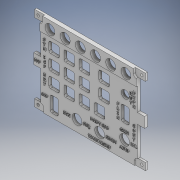
# Autodesk Inventor part: IPC Front Panel
Saved by Autodesk Inventor 2022 (Build 260153000, 153)
## iProperties
Created: 2021-12-31
Part Number: IPC Front Panel
Material: Generic
Document SubType Name: Modeling
Designer: solor
Density: 1 g/cm^3
Appearance: Default
Author: solor
Autodesk Inventor part; units mm, degrees
(part 1 of 2)
ref_plane "YZ Plane" through (0, 0, 0) normal (1, 0, 0) x (0, 1, 0)
ref_plane "XZ Plane" through (0, 0, 0) normal (0, 1, 0) x (-1, 0, 0)
ref_plane "XY Plane" through (0, 0, 0) normal (0, 0, 1) x (1, 0, 0)
sketch "Sketch1" plane through (0, 0, 0) normal (0, 0, 1) x (1, 0, 0)
  line L0 (0.0002, 13.311) -> (12.8002, 13.311) construction
  line L1 (12.8002, 13.311) -> (31.8502, 13.311) construction
  line L2 (31.8502, 13.311) -> (50.9002, 13.311) construction
  line L3 (50.9002, 13.311) -> (69.9502, 13.311) construction
  line L4 (69.9502, 13.311) -> (89.0002, 13.311) construction
  line L5 (89.0002, 13.311) -> (108.0502, 13.311) construction
  line L6 (-24.0572, 0) -> (-24.0572, -106) construction
  line L7 (0.0002, 13.311) -> (-8.9998, 13.311) construction
  line L8 (108.0502, 13.311) -> (120.8502, 13.311) construction
  line L9 (138.0271, 0) -> (138.0271, -10.03) construction
  line L10 (120.8502, 13.311) -> (129.8502, 13.311) construction
  line L11 (-9, 0) -> (-9, -9)
  line L12 (-9, -9) -> (-9, -46.5) construction
  line L13 (-9, -46.5) -> (-9, -59.5)
  line L14 (-9, -59.5) -> (-9, -97) construction
  line L15 (-9, -97) -> (-9, -106)
  line L16 (10, -106) -> (10, -100.81) construction
  line L17 (10, -100.81) -> (10, -81.47) construction
  line L18 (10, -81.47) -> (10, -75.06) construction
  line L19 (10, -75.06) -> (10, -61.92)
  line L20 (10, -61.92) -> (10, -56.04) construction
  line L21 (10, -56.04) -> (10, -42.9)
  line L22 (10, -42.9) -> (10, -37.02) construction
  line L23 (10, -37.02) -> (10, -23.88)
  line L24 (0, -23.88) -> (10, -23.88) construction
  line L25 (10, -23.88) -> (23.08, -23.88)
  line L26 (23.08, -23.88) -> (29.02, -23.88) construction
  line L27 (29.02, -23.88) -> (42.1, -23.88)
  line L28 (42.1, -23.88) -> (48.04, -23.88) construction
  line L29 (48.04, -23.88) -> (61.13, -23.88)
  line L30 (61.13, -23.88) -> (72.63, -23.88) construction
  line L31 (72.63, -23.88) -> (85.71, -23.88)
  line L32 (23.08, -23.88) -> (23.08, -37.02)
  line L33 (23.08, -37.02) -> (10, -37.02)
  line L34 (29.02, -23.88) -> (29.02, -37.02)
  line L35 (29.02, -37.02) -> (42.1, -37.02)
  line L36 (42.1, -37.02) -> (42.1, -23.88)
  line L37 (48.04, -23.88) -> (48.04, -37.02)
  line L38 (48.04, -37.02) -> (61.13, -37.02)
  line L39 (61.13, -37.02) -> (61.13, -23.88)
  line L40 (72.63, -23.88) -> (72.63, -37.02)
  line L41 (72.63, -37.02) -> (85.71, -37.02)
  line L42 (85.71, -37.02) -> (85.71, -23.88)
  line L43 (10, -42.9) -> (23.08, -42.9)
  line L44 (23.08, -42.9) -> (23.08, -56.04)
  line L45 (23.08, -56.04) -> (10, -56.04)
  line L46 (29.02, -42.9) -> (29.02, -56.04)
  line L47 (42.1, -56.04) -> (42.1, -42.9)
  line L48 (29.02, -56.04) -> (42.1, -56.04)
  line L49 (42.1, -42.9) -> (29.02, -42.9)
  line L50 (48.04, -42.9) -> (48.04, -56.04)
  line L51 (48.04, -56.04) -> (61.13, -56.04)
  line L52 (61.13, -56.04) -> (61.13, -42.9)
  line L53 (61.13, -42.9) -> (48.04, -42.9)
  line L54 (72.63, -42.9) -> (72.63, -56.04)
  line L55 (72.63, -56.04) -> (85.71, -56.04)
  line L56 (85.71, -56.04) -> (85.71, -42.9)
  line L57 (85.71, -42.9) -> (72.63, -42.9)
  line L58 (10, -61.92) -> (23.08, -61.92)
  line L59 (23.08, -61.92) -> (23.08, -75.06)
  line L60 (23.08, -75.06) -> (10, -75.06)
  line L61 (29.02, -61.92) -> (42.1, -61.92)
  line L62 (42.1, -61.92) -> (42.1, -75.06)
  line L63 (42.1, -75.06) -> (29.02, -75.06)
  line L64 (29.02, -75.06) -> (29.02, -61.92)
  line L65 (48.04, -61.92) -> (61.13, -61.92)
  line L66 (61.13, -61.92) -> (61.13, -75.06)
  line L67 (61.13, -75.06) -> (48.04, -75.06)
  line L68 (48.04, -75.06) -> (48.04, -61.92)
  line L69 (61.13, -61.92) -> (67.07, -61.92) construction
  line L70 (85.71, -49.47) -> (100.7, -49.47) construction
  line L71 (80.14, -61.92) -> (80.14, -75.06)
  line L72 (80.14, -75.06) -> (67.07, -75.06)
  line L73 (67.07, -75.06) -> (67.07, -61.92)
  line L74 (67.07, -61.92) -> (80.14, -61.92)
  circle A0 centre (12.8, -10.03) radius 6.22
  circle A1 centre (31.85, -10.03) radius 6.22
  circle A2 centre (50.9, -10.03) radius 6.22
  circle A3 centre (69.95, -10.03) radius 6.22
  circle A4 centre (89, -10.03) radius 6.22
  circle A5 centre (108.05, -10.03) radius 6.22
  line L75 (-9, -9) -> (0, -9)
  line L76 (0, -9) -> (0, -46.5)
  line L77 (0, -46.5) -> (-9, -46.5)
  line L78 (-9, -59.5) -> (0, -59.5)
  line L79 (0, -59.5) -> (0, -97)
  line L80 (0, -97) -> (-9, -97)
  line L81 (-9, 0) -> (129.8502, 0)
  line L82 (129.8502, -9) -> (120.8502, -9)
  line L83 (120.8502, -9) -> (120.8502, -46.5)
  line L84 (120.8502, -46.5) -> (129.8502, -46.5)
  line L85 (129.8502, -46.5) -> (129.8502, -59.5)
  line L86 (129.8502, -59.5) -> (120.8502, -59.5)
  line L87 (120.8502, -59.5) -> (120.8502, -97)
  line L88 (120.8502, -97) -> (129.8502, -97)
  line L89 (129.8502, -97) -> (129.8502, -106)
  line L90 (-9, -106) -> (129.8502, -106)
  line L91 (129.8502, 0) -> (129.8502, -9)
  line L92 (118.3416, -106) -> (118.3416, -84.37) construction
  line L93 (118.3416, -84.37) -> (118.3416, -66.16) construction
  line L94 (118.3416, -66.16) -> (118.3416, -46.82) construction
  circle A6 centre (104.8902, -84.37) radius 6.22
  line L95 (120.8502, -117.5908) -> (104.8902, -117.5908) construction
  line L96 (104.8902, -117.5908) -> (73.6502, -117.5908) construction
  line L97 (73.6502, -117.5908) -> (45.1902, -117.5908) construction
  line L98 (45.1902, -117.5908) -> (21.7302, -117.5908) construction
  line L99 (21.7302, -117.5908) -> (11.8502, -117.5908) construction
  line L100 (138.0271, -106) -> (138.0271, -92.18) construction
  circle A7 centre (73.6502, -92.18) radius 6.22
  circle A8 centre (45.1902, -92.18) radius 6.22
  line L101 (21.7302, -100.81) -> (21.7302, -81.47)
  line L102 (21.7302, -81.47) -> (11.8502, -81.47)
  line L103 (11.8502, -81.47) -> (11.8502, -100.81)
  line L104 (11.8502, -100.81) -> (21.7302, -100.81)
  line L105 (100.7, -46.82) -> (110.58, -46.82)
  line L106 (110.58, -46.82) -> (110.58, -66.16)
  line L107 (110.58, -66.16) -> (100.7, -66.16)
  line L108 (100.7, -66.16) -> (100.7, -46.82)
  line L109 (118.3416, -46.82) -> (118.3416, -34.66) construction
  line L110 (118.3416, -34.66) -> (118.3416, -18) construction
  line L111 (120.8502, -18) -> (0, -18)
  circle A9 centre (105.64, -34.66) radius 4.94
  point P0 (0, 0)
  dimension "d1" = 19.05
  dimension "d2" = 19.05
  dimension "d3" = 19.05
  dimension "d4" = 19.05
  dimension "d5" = 19.05
  dimension "d6" = 106
  dimension "d8" = 12.8
  dimension "d10" = 10.03
  dimension "d11" = 9
  dimension "d12" = 9
  dimension "d13" = 37.5
  dimension "d14" = 13
  dimension "d15" = 37.5
  dimension "d16" = 9
  dimension "d17" = 5.19
  dimension "d18" = 19.34
  dimension "d19" = 6.41
  dimension "d20" = 13.14
  dimension "d21" = 5.88
  dimension "d22" = 13.14
  dimension "d23" = 5.88
  dimension "d24" = 13.14
  dimension "d25" = 10
  dimension "d26" = 13.08
  dimension "d27" = 5.94
  dimension "d28" = 13.08
  dimension "d29" = 5.94
  dimension "d30" = 13.09
  dimension "d31" = 11.5
  dimension "d32" = 13.08
  dimension "d33" = 5.94
  dimension "d34" = 14.99
  dimension "d36" = 12.44
  dimension "d37" = 12.44
  dimension "d38" = 12.44
  dimension "d39" = 12.44
  dimension "d40" = 12.44
  dimension "d41" = 12.44
  dimension "d42" = 9
  dimension "d43" = 12.8
  dimension "d44" = 9
  dimension "d45" = 21.63
  dimension "d46" = 18.21
  dimension "d47" = 19.34
  dimension "d49" = 12.44
  dimension "d50" = 15.96
  dimension "d51" = 31.24
  dimension "d52" = 28.46
  dimension "d53" = 23.46
  dimension "d54" = 9.88
  dimension "d55" = 13.82
  dimension "d56" = 12.44
  dimension "d57" = 9.88
  dimension "d58" = 12.16
  dimension "d60" = 16.66
  dimension "d61" = 9.88
  constraints: 224 end point, 84 point on line, 31 perpendicular, 15 horizontal, 13 vertical, 10 centre point, 8 coincident, 4 parallel, 1 midpoint
  measures "d1" distance of L0.end L1.end
  measures "d2" distance of L1.end L2.end
  measures "d3" distance of L2.end L3.end
  measures "d4" distance of L3.end L4.end
  measures "d5" distance of L4.end L5.end
  measures "d6" distance of L6.start L6.end
  measures "d8" distance of L5.end L8.end
  measures "d10" distance of L9.start L9.end
  measures "d11" distance of L8.end L10.end
  measures "d12" distance of L11.start L11.end
  measures "d13" distance of L11.end L12.end
  measures "d14" distance of L12.end L13.end
  measures "d15" distance of L13.end L14.end
  measures "d16" distance of L14.end L15.end
  measures "d17" distance of L16.start L16.end
  measures "d18" distance of L16.end L17.end
  measures "d19" distance of L17.end L18.end
  measures "d20" distance of L18.end L19.end
  measures "d21" distance of L19.end L20.end
  measures "d22" distance of L20.end L21.end
  measures "d23" distance of L21.end L22.end
  measures "d24" distance of L22.end L23.end
  measures "d25" distance of L24.start L24.end
  measures "d26" distance of L24.end L25.end
  measures "d27" distance of L25.end L26.end
  measures "d28" distance of L26.end L27.end
  measures "d29" distance of L27.end L28.end
  measures "d30" distance of L28.end L29.end
  measures "d31" distance of L29.end L30.end
  measures "d32" distance of L30.end L31.end
  measures "d33" distance of L65.end L69.end
  measures "d34" distance of L70.start L70.end
  measures "d36" diameter of A0
  measures "d37" diameter of A1
  measures "d38" diameter of A2
  measures "d39" diameter of A3
  measures "d40" diameter of A4
  measures "d41" diameter of A5
  measures "d42" distance of L0.start L7.end
  measures "d43" distance of L0.start L0.end
  measures "d44" distance of L82.start L82.end
  measures "d45" distance of L92.start L92.end
  measures "d46" distance of L92.end L93.end
  measures "d47" distance of L93.end L94.end
  measures "d49" diameter of A6
  measures "d50" distance of L95.start L95.end
  measures "d51" distance of L95.end L96.end
  measures "d52" distance of L96.end L97.end
  measures "d53" distance of L97.end L98.end
  measures "d54" distance of L98.end L99.end
  measures "d55" distance of L100.start L100.end
  measures "d56" diameter of A7
  measures "d57" distance of L105.start L105.end
  measures "d58" distance of L94.end L109.end
  measures "d60" distance of L109.end L110.end
  measures "d61" diameter of A9
extrude "Extrusion1" add sketch "Sketch1" along normal blind 3.5 contours L111 L83 L84 L85 L86 L87 L88 L89 L90 L15 L80 L79 L78 L13 L77 L76
extrude "Extrusion2" add sketch "Sketch1" along normal blind 5 contours L81 L91 L82 L83 L111 L76 L75 L11
fillet "Fillet1" radius 2 4 edges at (10, -23.88, 1.75) (23.08, -23.88, 1.75) (10, -37.02, 1.75) (23.08, -37.02, 1.75)
fillet "Fillet2" radius 2 12 edges at (29.02, -23.88, 1.75) (29.02, -37.02, 1.75) (42.1, -37.02, 1.75) (42.1, -23.88, 1.75) (48.04, -23.88, 1.75) (48.04, -37.02, 1.75) (61.13, -37.02, 1.75) (61.13, -23.88, 1.75) (72.63, -23.88, 1.75) (72.63, -37.02, 1.75) (85.71, -37.02, 1.75) (85.71, -23.88, 1.75)
fillet "Fillet3" radius 2 20 edges at (10, -42.9, 1.75) (10, -56.04, 1.75) (23.08, -56.04, 1.75) (23.08, -42.9, 1.75) (29.02, -42.9, 1.75) (29.02, -56.04, 1.75) (42.1, -56.04, 1.75) (42.1, -42.9, 1.75) (48.04, -42.9, 1.75) (48.04, -56.04, 1.75) (61.13, -56.04, 1.75) (61.13, -42.9, 1.75) (72.63, -42.9, 1.75) (72.63, -56.04, 1.75) (85.71, -56.04, 1.75) (85.71, -42.9, 1.75) (100.7, -46.82, 1.75) (100.7, -66.16, 1.75) (110.58, -66.16, 1.75) (110.58, -46.82, 1.75)
fillet "Fillet4" radius 2 20 edges at (10, -75.06, 1.75) (10, -61.92, 1.75) (23.08, -61.92, 1.75) (23.08, -75.06, 1.75) (29.02, -75.06, 1.75) (29.02, -61.92, 1.75) (42.1, -61.92, 1.75) (42.1, -75.06, 1.75) (48.04, -75.06, 1.75) (48.04, -61.92, 1.75) (61.13, -61.92, 1.75) (61.13, -75.06, 1.75) (67.07, -75.06, 1.75) (67.07, -61.92, 1.75) (80.14, -75.06, 1.75) (80.14, -61.92, 1.75) (21.7302, -100.81, 1.75) (11.8502, -100.81, 1.75) (11.8502, -81.47, 1.75) (21.7302, -81.47, 1.75)
sketch "Sketch2" plane through (0, 0, 5) normal (0, 0, 1) x (1, 0, 0)
  line L0 (-9, -9) -> (0, -9) projected
  line L1 (3.5, -5.5828) -> (3.5, 0)
  line L2 (129.8502, 0) -> (-9, 0) projected
  arc A0 (0, -9) -> (3.501, -5.499) centre (0, -5.499) ccw
  line L3 (0, -9) -> (0, -5.499) construction
  line L4 (3.501, -5.499) -> (0, -5.499) construction
  line L5 (60.4251, 0) -> (60.4251, -11.5403)
  line L6 (-9, -106) -> (129.8502, -106) projected
  line L7 (-42.3083, 0) -> (-42.3083, -53)
  line L8 (-42.3083, -53) -> (-15.0047, -53)
  line L9 (3.5, 0) -> (-9, 0)
  line L10 (-9, 0) -> (-9, -9) projected
  line L11 (-9, 0) -> (-9, -9)
  line L12 (0, -9) -> (0, -46.5) projected
  line L13 (-9, -9) -> (0, -9)
  circle A1 centre (-4.5, -4.5) radius 1.65
  line L14 (129.8502, -9) -> (120.8502, -9)
  line L15 (117.3502, -5.5828) -> (117.3502, 0)
  arc A2 (117.3492, -5.499) -> (120.8502, -9) centre (120.8502, -5.499) ccw
  line L16 (163.1585, -53) -> (135.855, -53)
  line L17 (117.3502, 0) -> (129.8502, 0)
  line L18 (129.8502, 0) -> (129.8502, -9)
  circle A3 centre (125.3502, -4.5) radius 1.65
  line L19 (-9, -97) -> (0, -97)
  line L20 (3.5, -100.4172) -> (3.5, -106)
  line L21 (129.8502, -106) -> (-9, -106)
  arc A4 (3.501, -100.501) -> (0, -97) centre (0, -100.501) ccw
  line L22 (-9, -106) -> (-9, -97)
  circle A5 centre (-4.5, -101.5) radius 1.65
  circle A6 centre (125.3502, -101.5) radius 1.65
  line L23 (129.8502, -97) -> (120.8502, -97)
  line L24 (129.8502, -106) -> (129.8502, -97)
  line L25 (117.3502, -100.4172) -> (117.3502, -106)
  arc A7 (120.8502, -97) -> (117.3492, -100.501) centre (120.8502, -100.501) ccw
  point P0 (0, 0)
  dimension "d71" = 90
  dimension "d72" = 53
  dimension "d73" = 3.3
  constraints: 42 end point, 23 symmetric about line, 12 point on circle, 8 centre point, 3 point on line, 3 vertical, 2 collinear, 1 horizontal, 1 midpoint, 1 perpendicular, 1 tangent, 6 other
  measures "d71" angle of L3 L4
  measures "d72" distance of L7.start L7.end
  measures "d73" diameter of A1
extrude "Extrusion3" cut sketch "Sketch2" against normal blind 2.5
extrude "Extrusion4" cut sketch "Sketch2" against normal blind 18.1375 contours A1 | A3 | A5 | A6
sketch "Sketch3" plane through (0, 0, 3.5) normal (0, 0, 1) x (1, 0, 0)
  line L0 (3.5998, -42.9233) -> (6.4002, -42.9233) construction
  line L1 (6.4002, -42.9233) -> (6.4002, -56.0167) construction
  line L2 (6.4002, -56.0167) -> (3.5998, -56.0167) construction
  line L3 (3.5998, -56.0167) -> (3.5998, -42.9233) construction
  line L4 (3.4775, -61.9433) -> (6.5225, -61.9433) construction
  line L5 (6.5225, -61.9433) -> (6.5225, -75.0367) construction
  line L6 (6.5225, -75.0367) -> (3.4775, -75.0367) construction
  line L7 (3.4775, -75.0367) -> (3.4775, -61.9433) construction
  line L8 (-8.5522, -51.4107) -> (-0.4478, -51.4107) construction
  line L9 (-0.4478, -51.4107) -> (-0.4478, -54.5893) construction
  line L10 (-0.4478, -54.5893) -> (-8.5522, -54.5893) construction
  line L11 (-8.5522, -54.5893) -> (-8.5522, -51.4107) construction
  line L12 (0.9302, -84.0431) -> (9.0347, -84.0431) construction
  line L13 (9.0347, -84.0431) -> (9.0347, -87.2216) construction
  line L14 (9.0347, -87.2216) -> (0.9302, -87.2216) construction
  line L15 (0.9302, -87.2216) -> (0.9302, -84.0431) construction
  line L16 (28.3443, -90.655) -> (37.1902, -90.655) construction
  line L17 (37.1902, -90.655) -> (37.1902, -93.705) construction
  line L18 (37.1902, -93.705) -> (28.3443, -93.705) construction
  line L19 (28.3443, -93.705) -> (28.3443, -90.655) construction
  line L20 (53.1902, -90.1903) -> (61.6581, -90.1903) construction
  line L21 (61.6581, -90.1903) -> (61.6581, -94.1697) construction
  line L22 (61.6581, -94.1697) -> (53.1902, -94.1697) construction
  line L23 (53.1902, -94.1697) -> (53.1902, -90.1903) construction
  line L24 (62.1843, -80.3317) -> (85.1162, -80.3317) construction
  line L25 (85.1162, -80.3317) -> (85.1162, -84.18) construction
  line L26 (85.1162, -84.18) -> (62.1843, -84.18) construction
  line L27 (62.1843, -84.18) -> (62.1843, -80.3317) construction
  line L28 (59.5891, -100.18) -> (87.7114, -100.18) construction
  line L29 (87.7114, -100.18) -> (87.7114, -103.3388) construction
  line L30 (87.7114, -103.3388) -> (59.5891, -103.3388) construction
  line L31 (59.5891, -103.3388) -> (59.5891, -100.18) construction
  line L32 (81.6502, -90.5907) -> (94.9056, -90.5907) construction
  line L33 (94.9056, -90.5907) -> (94.9056, -93.7693) construction
  line L34 (94.9056, -93.7693) -> (81.6502, -93.7693) construction
  line L35 (81.6502, -93.7693) -> (81.6502, -90.5907) construction
  line L36 (99.2623, -73.1964) -> (110.5182, -73.1964) construction
  line L37 (110.5182, -73.1964) -> (110.5182, -76.37) construction
  line L38 (110.5182, -76.37) -> (99.2623, -76.37) construction
  line L39 (99.2623, -76.37) -> (99.2623, -73.1964) construction
  line L40 (99.0053, -92.37) -> (110.7752, -92.37) construction
  line L41 (110.7752, -92.37) -> (110.7752, -95.5485) construction
  line L42 (110.7752, -95.5485) -> (99.0053, -95.5485) construction
  line L43 (99.0053, -95.5485) -> (99.0053, -92.37) construction
  line L44 (112.8902, -82.845) -> (120.5202, -82.845) construction
  line L45 (120.5202, -82.845) -> (120.5202, -85.895) construction
  line L46 (120.5202, -85.895) -> (112.8902, -85.895) construction
  line L47 (112.8902, -85.895) -> (112.8902, -82.845) construction
  line L48 (115.4917, -61.3021) -> (118.7246, -61.3021) construction
  line L49 (118.7246, -61.3021) -> (118.7246, -79.4767) construction
  line L50 (118.7246, -79.4767) -> (115.4917, -79.4767) construction
  line L51 (115.4917, -79.4767) -> (115.4917, -61.3021) construction
  line L52 (95.6549, -47.4324) -> (98.7, -47.4324) construction
  line L53 (98.7, -47.4324) -> (98.7, -65.5476) construction
  line L54 (98.7, -65.5476) -> (95.6549, -65.5476) construction
  line L55 (95.6549, -65.5476) -> (95.6549, -47.4324) construction
  line L56 (115.64, -25.6024) -> (118.8161, -25.6024) construction
  line L57 (118.8161, -25.6024) -> (118.8161, -43.7176) construction
  line L58 (118.8161, -43.7176) -> (115.64, -43.7176) construction
  line L59 (115.64, -43.7176) -> (115.64, -25.6024) construction
  line L60 (111.64, -28.1133) -> (114.6851, -28.1133) construction
  line L61 (114.6851, -28.1133) -> (114.6851, -41.2067) construction
  line L62 (114.6851, -41.2067) -> (111.64, -41.2067) construction
  line L63 (111.64, -41.2067) -> (111.64, -28.1133) construction
  line L64 (10, -35.02) -> (10, -25.88) projected
  line L65 (0, -9) -> (0, -46.5) projected
  line L66 (0, -19.838) -> (10, -19.838)
  line L67 (3.1265, -23.8761) -> (6.8735, -23.8761) construction
  line L68 (6.8735, -23.8761) -> (6.8735, -37.0239) construction
  line L69 (6.8735, -37.0239) -> (3.1265, -37.0239) construction
  line L70 (3.1265, -37.0239) -> (3.1265, -23.8761) construction
  line L71 (10, -54.04) -> (10, -44.9) projected
  line L72 (10, -73.06) -> (10, -63.92) projected
  line L73 (-9, -59.5) -> (0, -59.5) projected
  line L74 (-9, -46.5) -> (-9, -59.5) projected
  circle A0 centre (45.1902, -92.18) radius 6.22 construction
  circle A1 centre (73.6502, -92.18) radius 6.22 construction
  line L75 (45.1902, -92.18) -> (37.1902, -92.18) construction
  line L76 (45.1902, -92.18) -> (53.1902, -92.18) construction
  line L77 (73.6502, -92.18) -> (73.6502, -84.18) construction
  line L78 (73.6502, -92.18) -> (81.6502, -92.18) construction
  line L79 (73.6502, -92.18) -> (73.6502, -100.18) construction
  circle A2 centre (104.8902, -84.37) radius 6.22 construction
  line L80 (104.8902, -84.37) -> (112.8902, -84.37) construction
  line L81 (104.8902, -84.37) -> (104.8902, -76.37) construction
  line L82 (104.8902, -84.37) -> (104.8902, -92.37) construction
  line L83 (100.7, -64.16) -> (100.7, -48.82) construction
  circle A3 centre (105.64, -34.66) radius 4.94 construction
  spline S0 degree 2 poles (-5.4602, -53) (-5.4602, -53.7415) (-6.2512, -54.5893) (-6.9383, -54.5893) knots 0 0 0 1 2 2 2
  spline S1 degree 2 poles (-6.9383, -54.5893) (-7.6279, -54.5893) (-8.4138, -53.7316) (-8.4138, -53) knots 0 0 0 1 2 2 2
  spline S2 degree 2 poles (-8.4138, -53) (-8.4138, -52.2659) (-7.6279, -51.4107) (-6.9383, -51.4107) knots 0 0 0 1 2 2 2
  spline S3 degree 2 poles (-6.9383, -51.4107) (-6.2512, -51.4107) (-5.4602, -52.261) (-5.4602, -53) knots 0 0 0 1 2 2 2
  spline S4 degree 2 poles (-6.2512, -53) (-6.2512, -52.7256) (-6.3624, -52.3425) (-6.4588, -52.2214) knots 0 0 0 1 2 2 2
  spline S5 degree 2 poles (-6.4588, -52.2214) (-6.5552, -52.0954) (-6.8023, -51.9866) (-6.9358, -51.9866) knots 0 0 0 1 2 2 2
  spline S6 degree 2 poles (-6.9358, -51.9866) (-7.0767, -51.9866) (-7.3065, -52.088) (-7.4128, -52.2165) knots 0 0 0 1 2 2 2
  spline S7 degree 2 poles (-7.4128, -52.2165) (-7.5067, -52.3351) (-7.6229, -52.7281) (-7.6229, -53) knots 0 0 0 1 2 2 2
  spline S8 degree 2 poles (-7.6229, -53) (-7.6229, -53.2818) (-7.5117, -53.6525) (-7.4153, -53.7786) knots 0 0 0 1 2 2 2
  spline S9 degree 2 poles (-7.4153, -53.7786) (-7.3189, -53.9046) (-7.0693, -54.0134) (-6.9358, -54.0134) knots 0 0 0 1 2 2 2
  spline S10 degree 2 poles (-6.9358, -54.0134) (-6.7999, -54.0134) (-6.5478, -53.8972) (-6.4563, -53.7736) knots 0 0 0 1 2 2 2
  spline S11 degree 2 poles (-6.4563, -53.7736) (-6.3574, -53.6402) (-6.2512, -53.2867) (-6.2512, -53) knots 0 0 0 1 2 2 2
  line L84 (-2.9639, -52.0558) -> (-4.2442, -52.0558)
  line L85 (-4.2442, -52.0558) -> (-4.2442, -52.6317)
  line L86 (-4.2442, -52.6317) -> (-3.0652, -52.6317)
  line L87 (-3.0652, -52.6317) -> (-3.0652, -53.2126)
  line L88 (-3.0652, -53.2126) -> (-4.2442, -53.2126)
  line L89 (-4.2442, -53.2126) -> (-4.2442, -54.525)
  line L90 (-4.2442, -54.525) -> (-5.0054, -54.525)
  line L91 (-5.0054, -54.525) -> (-5.0054, -51.475)
  line L92 (-5.0054, -51.475) -> (-2.9639, -51.475)
  line L93 (-2.9639, -51.475) -> (-2.9639, -52.0558)
  line L94 (-0.5268, -52.0558) -> (-1.8072, -52.0558)
  line L95 (-1.8072, -52.0558) -> (-1.8072, -52.6317)
  line L96 (-1.8072, -52.6317) -> (-0.6282, -52.6317)
  line L97 (-0.6282, -52.6317) -> (-0.6282, -53.2126)
  line L98 (-0.6282, -53.2126) -> (-1.8072, -53.2126)
  line L99 (-1.8072, -53.2126) -> (-1.8072, -54.525)
  line L100 (-1.8072, -54.525) -> (-2.5684, -54.525)
  line L101 (-2.5684, -54.525) -> (-2.5684, -51.475)
  line L102 (-2.5684, -51.475) -> (-0.5268, -51.475)
  line L103 (-0.5268, -51.475) -> (-0.5268, -52.0558)
  line L104 (5.4338, -45.9733) -> (3.7926, -45.9733)
  line L105 (3.7926, -45.9733) -> (3.7926, -45.4419)
  line L106 (3.7926, -45.4419) -> (4.2301, -45.4419)
  line L107 (4.2301, -45.4419) -> (4.2301, -43.4547)
  line L108 (4.2301, -43.4547) -> (3.7926, -43.4547)
  line L109 (3.7926, -43.4547) -> (3.7926, -42.9233)
  line L110 (3.7926, -42.9233) -> (5.4338, -42.9233)
  line L111 (5.4338, -42.9233) -> (5.4338, -43.4547)
  line L112 (5.4338, -43.4547) -> (4.9963, -43.4547)
  line L113 (4.9963, -43.4547) -> (4.9963, -45.4419)
  line L114 (4.9963, -45.4419) -> (5.4338, -45.4419)
  line L115 (5.4338, -45.4419) -> (5.4338, -45.9733)
  spline S12 degree 2 poles (5.2311, -51.0543) (4.544, -51.0543) (3.7382, -50.2238) (3.7382, -49.4725) knots 0 0 0 1 2 2 2
  spline S13 degree 2 poles (3.7382, -49.4725) (3.7382, -48.7483) (4.5465, -47.8857) (5.2336, -47.8857) knots 0 0 0 1 2 2 2
  spline S14 degree 2 poles (5.2336, -47.8857) (5.414, -47.8857) (5.7057, -47.9277) (5.8391, -47.9623) knots 0 0 0 1 2 2 2
  spline S15 degree 2 poles (5.8391, -47.9623) (5.9429, -47.9944) (6.1876, -48.1007) (6.2642, -48.1403) knots 0 0 0 1 2 2 2
  line L116 (6.2642, -48.1403) -> (6.2642, -48.8669)
  line L117 (6.2642, -48.8669) -> (6.1876, -48.8669)
  spline S16 degree 2 poles (6.1876, -48.8669) (6.1308, -48.8175) (5.9627, -48.6791) (5.8564, -48.6148) knots 0 0 0 1 2 2 2
  spline S17 degree 2 poles (5.8564, -48.6148) (5.7501, -48.5481) (5.4956, -48.4566) (5.3547, -48.4566) knots 0 0 0 1 2 2 2
  spline S18 degree 2 poles (5.3547, -48.4566) (5.1891, -48.4566) (4.9147, -48.5604) (4.7887, -48.6914) knots 0 0 0 1 2 2 2
  spline S19 degree 2 poles (4.7887, -48.6914) (4.675, -48.8076) (4.5292, -49.2055) (4.5292, -49.4749) knots 0 0 0 1 2 2 2
  spline S20 degree 2 poles (4.5292, -49.4749) (4.5292, -49.7592) (4.6799, -50.1472) (4.8035, -50.2659) knots 0 0 0 1 2 2 2
  spline S21 degree 2 poles (4.8035, -50.2659) (4.9221, -50.382) (5.2138, -50.4834) (5.3596, -50.4834) knots 0 0 0 1 2 2 2
  spline S22 degree 2 poles (5.3596, -50.4834) (5.5104, -50.4834) (5.7847, -50.382) (5.8787, -50.3202) knots 0 0 0 1 2 2 2
  spline S23 degree 2 poles (5.8787, -50.3202) (5.9825, -50.2585) (6.1382, -50.1275) (6.195, -50.0756) knots 0 0 0 1 2 2 2
  line L118 (6.195, -50.0756) -> (6.2642, -50.0756)
  line L119 (6.2642, -50.0756) -> (6.2642, -50.7923)
  spline S24 degree 2 poles (6.2642, -50.7923) (6.1802, -50.8319) (5.9602, -50.9307) (5.8416, -50.9653) knots 0 0 0 1 2 2 2
  spline S25 degree 2 poles (5.8416, -50.9653) (5.6982, -51.0098) (5.4486, -51.0543) (5.2311, -51.0543) knots 0 0 0 1 2 2 2
  spline S26 degree 2 poles (6.2618, -53.9282) (6.2618, -54.1408) (6.1258, -54.5263) (5.9998, -54.6549) knots 0 0 0 1 2 2 2
  spline S27 degree 2 poles (5.9998, -54.6549) (5.9232, -54.7364) (5.7353, -54.8699) (5.6241, -54.9169) knots 0 0 0 1 2 2 2
  spline S28 degree 2 poles (5.6241, -54.9169) (5.5104, -54.9638) (5.2459, -55.0182) (5.0828, -55.0182) knots 0 0 0 1 2 2 2
  line L120 (5.0828, -55.0182) -> (4.6824, -55.0182)
  line L121 (4.6824, -55.0182) -> (4.6824, -56.0167)
  line L122 (4.6824, -56.0167) -> (3.9162, -56.0167)
  line L123 (3.9162, -56.0167) -> (3.9162, -52.9667)
  line L124 (3.9162, -52.9667) -> (5.1001, -52.9667)
  spline S29 degree 2 poles (5.1001, -52.9667) (5.3621, -52.9667) (5.7452, -53.0631) (5.9009, -53.1669) knots 0 0 0 1 2 2 2
  spline S30 degree 2 poles (5.9009, -53.1669) (6.0739, -53.2831) (6.2618, -53.6637) (6.2618, -53.9282) knots 0 0 0 1 2 2 2
  spline S31 degree 2 poles (5.4758, -53.948) (5.4758, -53.817) (5.3522, -53.6316) (5.2682, -53.597) knots 0 0 0 1 2 2 2
  spline S32 degree 2 poles (5.2682, -53.597) (5.1594, -53.5501) (4.9617, -53.5352) (4.7911, -53.5352) knots 0 0 0 1 2 2 2
  line L125 (4.7911, -53.5352) -> (4.6824, -53.5352)
  line L126 (4.6824, -53.5352) -> (4.6824, -54.4497)
  line L127 (4.6824, -54.4497) -> (4.7368, -54.4497)
  spline S33 degree 2 poles (4.7368, -54.4497) (4.8431, -54.4497) (5.0358, -54.4448) (5.1075, -54.4324) knots 0 0 0 1 2 2 2
  spline S34 degree 2 poles (5.1075, -54.4324) (5.1693, -54.4225) (5.3052, -54.3632) (5.3423, -54.3261) knots 0 0 0 1 2 2 2
  spline S35 degree 2 poles (5.3423, -54.3261) (5.4214, -54.252) (5.4758, -54.0864) (5.4758, -53.948) knots 0 0 0 1 2 2 2
  spline S36 degree 2 poles (4.3846, -27.0348) (4.0336, -27.0348) (3.5047, -26.8989) (3.2773, -26.8) knots 0 0 0 1 2 2 2
  line L128 (3.2773, -26.8) -> (3.2773, -26.0734)
  line L129 (3.2773, -26.0734) -> (3.3465, -26.0734)
  spline S37 degree 2 poles (3.3465, -26.0734) (3.5763, -26.2686) (4.1275, -26.4787) (4.387, -26.4787) knots 0 0 0 1 2 2 2
  spline S38 degree 2 poles (4.387, -26.4787) (4.4538, -26.4787) (4.6688, -26.449) (4.7331, -26.4194) knots 0 0 0 1 2 2 2
  spline S39 degree 2 poles (4.7331, -26.4194) (4.8122, -26.3848) (4.9234, -26.2587) (4.9234, -26.1574) knots 0 0 0 1 2 2 2
  spline S40 degree 2 poles (4.9234, -26.1574) (4.9234, -26.0412) (4.7429, -25.8979) (4.6194, -25.8657) knots 0 0 0 1 2 2 2
  spline S41 degree 2 poles (4.6194, -25.8657) (4.4637, -25.8237) (4.1102, -25.752) (3.9545, -25.6977) knots 0 0 0 1 2 2 2
  spline S42 degree 2 poles (3.9545, -25.6977) (3.6011, -25.5741) (3.2946, -25.1514) (3.2946, -24.8351) knots 0 0 0 1 2 2 2
  spline S43 degree 2 poles (3.2946, -24.8351) (3.2946, -24.4075) (4.0188, -23.8761) (4.5625, -23.8761) knots 0 0 0 1 2 2 2
  spline S44 degree 2 poles (4.5625, -23.8761) (4.8344, -23.8761) (5.3732, -23.9873) (5.5858, -24.0812) knots 0 0 0 1 2 2 2
  line L130 (5.5858, -24.0812) -> (5.5858, -24.7782)
  line L131 (5.5858, -24.7782) -> (5.519, -24.7782)
  spline S45 degree 2 poles (5.519, -24.7782) (5.3485, -24.6324) (4.8591, -24.4322) (4.6021, -24.4322) knots 0 0 0 1 2 2 2
  spline S46 degree 2 poles (4.6021, -24.4322) (4.5007, -24.4322) (4.3425, -24.4618) (4.2536, -24.5014) knots 0 0 0 1 2 2 2
  spline S47 degree 2 poles (4.2536, -24.5014) (4.1819, -24.5335) (4.0781, -24.662) (4.0781, -24.7411) knots 0 0 0 1 2 2 2
  spline S48 degree 2 poles (4.0781, -24.7411) (4.0781, -24.8598) (4.2437, -24.9957) (4.481, -25.0501) knots 0 0 0 1 2 2 2
  spline S49 degree 2 poles (4.481, -25.0501) (4.6342, -25.0847) (4.9184, -25.1514) (5.0816, -25.2083) knots 0 0 0 1 2 2 2
  spline S50 degree 2 poles (5.0816, -25.2083) (5.3979, -25.3244) (5.7069, -25.71) (5.7069, -26.0264) knots 0 0 0 1 2 2 2
  spline S51 degree 2 poles (5.7069, -26.0264) (5.7069, -26.4812) (4.9926, -27.0348) (4.3846, -27.0348) knots 0 0 0 1 2 2 2
  line L132 (5.9788, -28.9522) -> (4.9259, -30.7293)
  line L133 (4.9259, -30.7293) -> (4.9259, -32.0022)
  line L134 (4.9259, -32.0022) -> (4.1596, -32.0022)
  line L135 (4.1596, -32.0022) -> (4.1596, -30.7664)
  line L136 (4.1596, -30.7664) -> (3.0894, -28.9522)
  line L137 (3.0894, -28.9522) -> (3.9619, -28.9522)
  line L138 (3.9619, -28.9522) -> (4.5576, -30.0397)
  line L139 (4.5576, -30.0397) -> (5.1335, -28.9522)
  line L140 (5.1335, -28.9522) -> (5.9788, -28.9522)
  line L141 (6.5571, -37.0239) -> (5.7959, -37.0239)
  line L142 (5.7959, -37.0239) -> (5.7959, -35.0021)
  line L143 (5.7959, -35.0021) -> (5.2422, -36.3072)
  line L144 (5.2422, -36.3072) -> (4.7182, -36.3072)
  line L145 (4.7182, -36.3072) -> (4.1646, -35.0021)
  line L146 (4.1646, -35.0021) -> (4.1646, -37.0239)
  line L147 (4.1646, -37.0239) -> (3.4429, -37.0239)
  line L148 (3.4429, -37.0239) -> (3.4429, -33.9739)
  line L149 (3.4429, -33.9739) -> (4.3252, -33.9739)
  line L150 (4.3252, -33.9739) -> (5.0025, -35.4792)
  line L151 (5.0025, -35.4792) -> (5.6748, -33.9739)
  line L152 (5.6748, -33.9739) -> (6.5571, -33.9739)
  line L153 (6.5571, -33.9739) -> (6.5571, -37.0239)
  spline S52 degree 2 poles (6.2309, -64.059) (6.2309, -64.2864) (6.0579, -64.6299) (5.9145, -64.7436) knots 0 0 0 1 2 2 2
  spline S53 degree 2 poles (5.9145, -64.7436) (5.7415, -64.8796) (5.3312, -64.9933) (5.0124, -64.9933) knots 0 0 0 1 2 2 2
  line L154 (5.0124, -64.9933) -> (3.7938, -64.9933)
  line L155 (3.7938, -64.9933) -> (3.7938, -61.9433)
  line L156 (3.7938, -61.9433) -> (4.869, -61.9433)
  spline S54 degree 2 poles (4.869, -61.9433) (5.2051, -61.9433) (5.5512, -61.9952) (5.7019, -62.0767) knots 0 0 0 1 2 2 2
  spline S55 degree 2 poles (5.7019, -62.0767) (5.8675, -62.1632) (6.0282, -62.4598) (6.0282, -62.6526) knots 0 0 0 1 2 2 2
  spline S56 degree 2 poles (6.0282, -62.6526) (6.0282, -62.8751) (5.8058, -63.2236) (5.608, -63.3051) knots 0 0 0 1 2 2 2
  line L157 (5.608, -63.3051) -> (5.608, -63.32)
  spline S57 degree 2 poles (5.608, -63.32) (5.8923, -63.3793) (6.2309, -63.7476) (6.2309, -64.059) knots 0 0 0 1 2 2 2
  spline S58 degree 2 poles (5.44, -64.0466) (5.44, -63.9033) (5.3263, -63.7426) (5.2126, -63.7006) knots 0 0 0 1 2 2 2
  spline S59 degree 2 poles (5.2126, -63.7006) (5.1434, -63.6734) (4.8987, -63.6685) (4.696, -63.6685) knots 0 0 0 1 2 2 2
  line L158 (4.696, -63.6685) -> (4.5551, -63.6685)
  line L159 (4.5551, -63.6685) -> (4.5551, -64.4371)
  line L160 (4.5551, -64.4371) -> (4.5971, -64.4371)
  spline S60 degree 2 poles (4.5971, -64.4371) (4.8937, -64.4371) (5.1211, -64.4297) (5.2397, -64.3778) knots 0 0 0 1 2 2 2
  spline S61 degree 2 poles (5.2397, -64.3778) (5.3436, -64.3309) (5.44, -64.1578) (5.44, -64.0466) knots 0 0 0 1 2 2 2
  spline S62 degree 2 poles (5.2496, -62.8034) (5.2496, -62.7292) (5.173, -62.5735) (5.0939, -62.5389) knots 0 0 0 1 2 2 2
  spline S63 degree 2 poles (5.0939, -62.5389) (5.0198, -62.5043) (4.8122, -62.4994) (4.607, -62.4994) knots 0 0 0 1 2 2 2
  line L161 (4.607, -62.4994) -> (4.5551, -62.4994)
  line L162 (4.5551, -62.4994) -> (4.5551, -63.1469)
  line L163 (4.5551, -63.1469) -> (4.6515, -63.1469)
  spline S64 degree 2 poles (4.6515, -63.1469) (4.8468, -63.1469) (5.0049, -63.1395) (5.089, -63.1) knots 0 0 0 1 2 2 2
  spline S65 degree 2 poles (5.089, -63.1) (5.1804, -63.0555) (5.2496, -62.9047) (5.2496, -62.8034) knots 0 0 0 1 2 2 2
  line L164 (6.6115, -70.015) -> (5.6797, -70.015)
  line L165 (5.6797, -70.015) -> (4.8319, -68.8953)
  line L166 (4.8319, -68.8953) -> (4.5551, -68.8953)
  line L167 (4.5551, -68.8953) -> (4.5551, -70.015)
  line L168 (4.5551, -70.015) -> (3.7938, -70.015)
  line L169 (3.7938, -70.015) -> (3.7938, -66.965)
  line L170 (3.7938, -66.965) -> (5.0198, -66.965)
  spline S66 degree 2 poles (5.0198, -66.965) (5.2744, -66.965) (5.65, -67.0293) (5.8107, -67.1281) knots 0 0 0 1 2 2 2
  spline S67 degree 2 poles (5.8107, -67.1281) (5.9738, -67.2319) (6.1666, -67.5557) (6.1666, -67.8029) knots 0 0 0 1 2 2 2
  spline S68 degree 2 poles (6.1666, -67.8029) (6.1666, -68.1514) (5.8502, -68.5889) (5.5858, -68.7174) knots 0 0 0 1 2 2 2
  line L171 (5.5858, -68.7174) -> (6.6115, -70.015)
  spline S69 degree 2 poles (5.3806, -67.8993) (5.3806, -67.7831) (5.2917, -67.6175) (5.1903, -67.573) knots 0 0 0 1 2 2 2
  spline S70 degree 2 poles (5.1903, -67.573) (5.1186, -67.5434) (4.9432, -67.5261) (4.8122, -67.5261) knots 0 0 0 1 2 2 2
  line L172 (4.8122, -67.5261) -> (4.5551, -67.5261)
  line L173 (4.5551, -67.5261) -> (4.5551, -68.3466)
  line L174 (4.5551, -68.3466) -> (4.7751, -68.3466)
  spline S71 degree 2 poles (4.7751, -68.3466) (4.9333, -68.3466) (5.1582, -68.3071) (5.2348, -68.2453) knots 0 0 0 1 2 2 2
  spline S72 degree 2 poles (5.2348, -68.2453) (5.309, -68.186) (5.3806, -68.0278) (5.3806, -67.8993) knots 0 0 0 1 2 2 2
  line L175 (4.3796, -75.0367) -> (4.3796, -72.5676)
  line L176 (4.3796, -72.5676) -> (3.4775, -72.5676)
  line L177 (3.4775, -72.5676) -> (3.4775, -71.9867)
  line L178 (3.4775, -71.9867) -> (6.048, -71.9867)
  line L179 (6.048, -71.9867) -> (6.048, -72.5676)
  line L180 (6.048, -72.5676) -> (5.1458, -72.5676)
  line L181 (5.1458, -72.5676) -> (5.1458, -75.0367)
  line L182 (5.1458, -75.0367) -> (4.3796, -75.0367)
  spline S73 degree 2 poles (4.0222, -85.6324) (4.0222, -86.3739) (3.2313, -87.2216) (2.5442, -87.2216) knots 0 0 0 1 2 2 2
  spline S74 degree 2 poles (2.5442, -87.2216) (1.8546, -87.2216) (1.0686, -86.364) (1.0686, -85.6324) knots 0 0 0 1 2 2 2
  spline S75 degree 2 poles (1.0686, -85.6324) (1.0686, -84.8983) (1.8546, -84.0431) (2.5442, -84.0431) knots 0 0 0 1 2 2 2
  spline S76 degree 2 poles (2.5442, -84.0431) (3.2313, -84.0431) (4.0222, -84.8934) (4.0222, -85.6324) knots 0 0 0 1 2 2 2
  spline S77 degree 2 poles (3.2313, -85.6324) (3.2313, -85.358) (3.1201, -84.9749) (3.0237, -84.8538) knots 0 0 0 1 2 2 2
  spline S78 degree 2 poles (3.0237, -84.8538) (2.9273, -84.7278) (2.6801, -84.619) (2.5466, -84.619) knots 0 0 0 1 2 2 2
  spline S79 degree 2 poles (2.5466, -84.619) (2.4058, -84.619) (2.1759, -84.7203) (2.0696, -84.8489) knots 0 0 0 1 2 2 2
  spline S80 degree 2 poles (2.0696, -84.8489) (1.9757, -84.9675) (1.8595, -85.3605) (1.8595, -85.6324) knots 0 0 0 1 2 2 2
  spline S81 degree 2 poles (1.8595, -85.6324) (1.8595, -85.9141) (1.9707, -86.2849) (2.0671, -86.4109) knots 0 0 0 1 2 2 2
  spline S82 degree 2 poles (2.0671, -86.4109) (2.1635, -86.537) (2.4132, -86.6457) (2.5466, -86.6457) knots 0 0 0 1 2 2 2
  spline S83 degree 2 poles (2.5466, -86.6457) (2.6826, -86.6457) (2.9347, -86.5296) (3.0261, -86.406) knots 0 0 0 1 2 2 2
  spline S84 degree 2 poles (3.0261, -86.406) (3.125, -86.2725) (3.2313, -85.9191) (3.2313, -85.6324) knots 0 0 0 1 2 2 2
  line L183 (6.5186, -84.6882) -> (5.2382, -84.6882)
  line L184 (5.2382, -84.6882) -> (5.2382, -85.2641)
  line L185 (5.2382, -85.2641) -> (6.4172, -85.2641)
  line L186 (6.4172, -85.2641) -> (6.4172, -85.8449)
  line L187 (6.4172, -85.8449) -> (5.2382, -85.8449)
  line L188 (5.2382, -85.8449) -> (5.2382, -87.1574)
  line L189 (5.2382, -87.1574) -> (4.477, -87.1574)
  line L190 (4.477, -87.1574) -> (4.477, -84.1074)
  line L191 (4.477, -84.1074) -> (6.5186, -84.1074)
  line L192 (6.5186, -84.1074) -> (6.5186, -84.6882)
  line L193 (8.9556, -84.6882) -> (7.6753, -84.6882)
  line L194 (7.6753, -84.6882) -> (7.6753, -85.2641)
  line L195 (7.6753, -85.2641) -> (8.8543, -85.2641)
  line L196 (8.8543, -85.2641) -> (8.8543, -85.8449)
  line L197 (8.8543, -85.8449) -> (7.6753, -85.8449)
  line L198 (7.6753, -85.8449) -> (7.6753, -87.1574)
  line L199 (7.6753, -87.1574) -> (6.914, -87.1574)
  line L200 (6.914, -87.1574) -> (6.914, -84.1074)
  line L201 (6.914, -84.1074) -> (8.9556, -84.1074)
  line L202 (8.9556, -84.1074) -> (8.9556, -84.6882)
  line L203 (31.4783, -93.705) -> (30.5465, -93.705)
  line L204 (30.5465, -93.705) -> (29.6987, -92.5853)
  line L205 (29.6987, -92.5853) -> (29.4219, -92.5853)
  line L206 (29.4219, -92.5853) -> (29.4219, -93.705)
  line L207 (29.4219, -93.705) -> (28.6606, -93.705)
  line L208 (28.6606, -93.705) -> (28.6606, -90.655)
  line L209 (28.6606, -90.655) -> (29.8866, -90.655)
  spline S85 degree 2 poles (29.8866, -90.655) (30.1411, -90.655) (30.5168, -90.7193) (30.6775, -90.8181) knots 0 0 0 1 2 2 2
  spline S86 degree 2 poles (30.6775, -90.8181) (30.8406, -90.9219) (31.0334, -91.2457) (31.0334, -91.4929) knots 0 0 0 1 2 2 2
  spline S87 degree 2 poles (31.0334, -91.4929) (31.0334, -91.8414) (30.717, -92.2789) (30.4526, -92.4074) knots 0 0 0 1 2 2 2
  line L210 (30.4526, -92.4074) -> (31.4783, -93.705)
  spline S88 degree 2 poles (30.2474, -91.5893) (30.2474, -91.4731) (30.1584, -91.3075) (30.0571, -91.263) knots 0 0 0 1 2 2 2
  spline S89 degree 2 poles (30.0571, -91.263) (29.9854, -91.2334) (29.8099, -91.2161) (29.6789, -91.2161) knots 0 0 0 1 2 2 2
  line L211 (29.6789, -91.2161) -> (29.4219, -91.2161)
  line L212 (29.4219, -91.2161) -> (29.4219, -92.0366)
  line L213 (29.4219, -92.0366) -> (29.6419, -92.0366)
  spline S90 degree 2 poles (29.6419, -92.0366) (29.8001, -92.0366) (30.025, -91.9971) (30.1016, -91.9353) knots 0 0 0 1 2 2 2
  spline S91 degree 2 poles (30.1016, -91.9353) (30.1757, -91.876) (30.2474, -91.7178) (30.2474, -91.5893) knots 0 0 0 1 2 2 2
  line L214 (32.2915, -93.705) -> (32.2915, -91.2358)
  line L215 (32.2915, -91.2358) -> (31.3893, -91.2358)
  line L216 (31.3893, -91.2358) -> (31.3893, -90.655)
  line L217 (31.3893, -90.655) -> (33.9598, -90.655)
  line L218 (33.9598, -90.655) -> (33.9598, -91.2358)
  line L219 (33.9598, -91.2358) -> (33.0577, -91.2358)
  line L220 (33.0577, -91.2358) -> (33.0577, -93.705)
  line L221 (33.0577, -93.705) -> (32.2915, -93.705)
  line L222 (36.8862, -93.705) -> (36.1497, -93.705)
  line L223 (36.1497, -93.705) -> (34.9732, -91.5794)
  line L224 (34.9732, -91.5794) -> (34.9732, -93.705)
  line L225 (34.9732, -93.705) -> (34.2737, -93.705)
  line L226 (34.2737, -93.705) -> (34.2737, -90.655)
  line L227 (34.2737, -90.655) -> (35.2129, -90.655)
  line L228 (35.2129, -90.655) -> (36.1868, -92.4024)
  line L229 (36.1868, -92.4024) -> (36.1868, -90.655)
  line L230 (36.1868, -90.655) -> (36.8862, -90.655)
  line L231 (36.8862, -90.655) -> (36.8862, -93.705)
  spline S92 degree 2 poles (54.4483, -93.359) (54.0973, -93.359) (53.5684, -93.223) (53.341, -93.1242) knots 0 0 0 1 2 2 2
  line L232 (53.341, -93.1242) -> (53.341, -92.3975)
  line L233 (53.341, -92.3975) -> (53.4102, -92.3975)
  spline S93 degree 2 poles (53.4102, -92.3975) (53.6401, -92.5928) (54.1913, -92.8029) (54.4508, -92.8029) knots 0 0 0 1 2 2 2
  spline S94 degree 2 poles (54.4508, -92.8029) (54.5175, -92.8029) (54.7325, -92.7732) (54.7968, -92.7435) knots 0 0 0 1 2 2 2
  spline S95 degree 2 poles (54.7968, -92.7435) (54.8759, -92.7089) (54.9871, -92.5829) (54.9871, -92.4815) knots 0 0 0 1 2 2 2
  spline S96 degree 2 poles (54.9871, -92.4815) (54.9871, -92.3654) (54.8067, -92.222) (54.6831, -92.1899) knots 0 0 0 1 2 2 2
  spline S97 degree 2 poles (54.6831, -92.1899) (54.5274, -92.1479) (54.174, -92.0762) (54.0182, -92.0218) knots 0 0 0 1 2 2 2
  spline S98 degree 2 poles (54.0182, -92.0218) (53.6648, -91.8982) (53.3583, -91.4756) (53.3583, -91.1592) knots 0 0 0 1 2 2 2
  spline S99 degree 2 poles (53.3583, -91.1592) (53.3583, -90.7316) (54.0825, -90.2002) (54.6263, -90.2002) knots 0 0 0 1 2 2 2
  spline S100 degree 2 poles (54.6263, -90.2002) (54.8981, -90.2002) (55.437, -90.3114) (55.6495, -90.4054) knots 0 0 0 1 2 2 2
  line L234 (55.6495, -90.4054) -> (55.6495, -91.1024)
  line L235 (55.6495, -91.1024) -> (55.5828, -91.1024)
  spline S101 degree 2 poles (55.5828, -91.1024) (55.4122, -90.9565) (54.9229, -90.7563) (54.6658, -90.7563) knots 0 0 0 1 2 2 2
  spline S102 degree 2 poles (54.6658, -90.7563) (54.5645, -90.7563) (54.4063, -90.786) (54.3173, -90.8255) knots 0 0 0 1 2 2 2
  spline S103 degree 2 poles (54.3173, -90.8255) (54.2456, -90.8577) (54.1418, -90.9862) (54.1418, -91.0653) knots 0 0 0 1 2 2 2
  spline S104 degree 2 poles (54.1418, -91.0653) (54.1418, -91.1839) (54.3074, -91.3199) (54.5447, -91.3742) knots 0 0 0 1 2 2 2
  spline S105 degree 2 poles (54.5447, -91.3742) (54.6979, -91.4088) (54.9822, -91.4756) (55.1453, -91.5324) knots 0 0 0 1 2 2 2
  spline S106 degree 2 poles (55.1453, -91.5324) (55.4617, -91.6486) (55.7706, -92.0342) (55.7706, -92.3505) knots 0 0 0 1 2 2 2
  spline S107 degree 2 poles (55.7706, -92.3505) (55.7706, -92.8053) (55.0563, -93.359) (54.4483, -93.359) knots 0 0 0 1 2 2 2
  line L236 (56.1636, -93.3046) -> (56.1636, -90.2546)
  line L237 (56.1636, -90.2546) -> (58.225, -90.2546)
  line L238 (58.225, -90.2546) -> (58.225, -90.8354)
  line L239 (58.225, -90.8354) -> (56.9249, -90.8354)
  line L240 (56.9249, -90.8354) -> (56.9249, -91.3718)
  line L241 (56.9249, -91.3718) -> (58.1236, -91.3718)
  line L242 (58.1236, -91.3718) -> (58.1236, -91.9526)
  line L243 (58.1236, -91.9526) -> (56.9249, -91.9526)
  line L244 (56.9249, -91.9526) -> (56.9249, -92.7238)
  line L245 (56.9249, -92.7238) -> (58.225, -92.7238)
  line L246 (58.225, -92.7238) -> (58.225, -93.3046)
  line L247 (58.225, -93.3046) -> (56.1636, -93.3046)
  spline S108 degree 2 poles (61.5147, -94.1103) (61.3911, -94.14) (61.144, -94.1697) (60.8795, -94.1697) knots 0 0 0 1 2 2 2
  spline S109 degree 2 poles (60.8795, -94.1697) (60.6398, -94.1697) (60.3011, -94.0486) (60.1875, -93.9373) knots 0 0 0 1 2 2 2
  spline S110 degree 2 poles (60.1875, -93.9373) (60.0762, -93.8286) (59.9625, -93.532) (59.9551, -93.359) knots 0 0 0 1 2 2 2
  spline S111 degree 2 poles (59.9551, -93.359) (59.31, -93.3293) (58.5661, -92.4914) (58.5661, -91.7796) knots 0 0 0 1 2 2 2
  spline S112 degree 2 poles (58.5661, -91.7796) (58.5661, -91.0455) (59.352, -90.1903) (60.0416, -90.1903) knots 0 0 0 1 2 2 2
  spline S113 degree 2 poles (60.0416, -90.1903) (60.7287, -90.1903) (61.5197, -91.0406) (61.5197, -91.7796) knots 0 0 0 1 2 2 2
  spline S114 degree 2 poles (61.5197, -91.7796) (61.5197, -92.3184) (61.0723, -93.0896) (60.662, -93.2527) knots 0 0 0 1 2 2 2
  spline S115 degree 2 poles (60.662, -93.2527) (60.6669, -93.4776) (60.8573, -93.6482) (61.0945, -93.6482) knots 0 0 0 1 2 2 2
  spline S116 degree 2 poles (61.0945, -93.6482) (61.1885, -93.6482) (61.3936, -93.5938) (61.4381, -93.5691) knots 0 0 0 1 2 2 2
  line L248 (61.4381, -93.5691) -> (61.5147, -93.5691)
  line L249 (61.5147, -93.5691) -> (61.5147, -94.1103)
  spline S117 degree 2 poles (60.5236, -92.5507) (60.6225, -92.4173) (60.7287, -92.0638) (60.7287, -91.7771) knots 0 0 0 1 2 2 2
  spline S118 degree 2 poles (60.7287, -91.7771) (60.7287, -91.5052) (60.6175, -91.1221) (60.5211, -90.9986) knots 0 0 0 1 2 2 2
  spline S119 degree 2 poles (60.5211, -90.9986) (60.4247, -90.875) (60.1776, -90.7662) (60.0441, -90.7662) knots 0 0 0 1 2 2 2
  spline S120 degree 2 poles (60.0441, -90.7662) (59.9032, -90.7662) (59.6733, -90.8676) (59.5671, -90.9961) knots 0 0 0 1 2 2 2
  spline S121 degree 2 poles (59.5671, -90.9961) (59.4731, -91.1147) (59.357, -91.5077) (59.357, -91.7796) knots 0 0 0 1 2 2 2
  spline S122 degree 2 poles (59.357, -91.7796) (59.357, -92.0589) (59.4682, -92.4296) (59.5646, -92.5557) knots 0 0 0 1 2 2 2
  spline S123 degree 2 poles (59.5646, -92.5557) (59.661, -92.6817) (59.9106, -92.7905) (60.0441, -92.7905) knots 0 0 0 1 2 2 2
  spline S124 degree 2 poles (60.0441, -92.7905) (60.18, -92.7905) (60.4321, -92.6743) (60.5236, -92.5507) knots 0 0 0 1 2 2 2
  spline S125 degree 2 poles (65.222, -81.9951) (65.222, -82.4227) (64.8487, -83.095) (64.5645, -83.2754) knots 0 0 0 1 2 2 2
  spline S126 degree 2 poles (64.5645, -83.2754) (64.3272, -83.4286) (63.7686, -83.5176) (63.4547, -83.5176) knots 0 0 0 1 2 2 2
  line L250 (63.4547, -83.5176) -> (62.5007, -83.5176)
  line L251 (62.5007, -83.5176) -> (62.5007, -80.4676)
  line L252 (62.5007, -80.4676) -> (63.4449, -80.4676)
  spline S127 degree 2 poles (63.4449, -80.4676) (63.7662, -80.4676) (64.3272, -80.5492) (64.5744, -80.7074) knots 0 0 0 1 2 2 2
  spline S128 degree 2 poles (64.5744, -80.7074) (64.8735, -80.9001) (65.222, -81.5526) (65.222, -81.9951) knots 0 0 0 1 2 2 2
  spline S129 degree 2 poles (64.436, -81.9901) (64.436, -81.6886) (64.2284, -81.2585) (64.0158, -81.1374) knots 0 0 0 1 2 2 2
  spline S130 degree 2 poles (64.0158, -81.1374) (63.8601, -81.0534) (63.519, -81.0361) (63.2817, -81.0361) knots 0 0 0 1 2 2 2
  line L253 (63.2817, -81.0361) -> (63.2669, -81.0361)
  line L254 (63.2669, -81.0361) -> (63.2669, -82.9467)
  line L255 (63.2669, -82.9467) -> (63.2817, -82.9467)
  spline S131 degree 2 poles (63.2817, -82.9467) (63.5388, -82.9467) (63.8922, -82.9294) (64.0529, -82.828) knots 0 0 0 1 2 2 2
  spline S132 degree 2 poles (64.0529, -82.828) (64.2407, -82.7094) (64.436, -82.2917) (64.436, -81.9901) knots 0 0 0 1 2 2 2
  line L256 (68.4944, -83.5176) -> (67.5626, -83.5176)
  line L257 (67.5626, -83.5176) -> (66.7148, -82.3979)
  line L258 (66.7148, -82.3979) -> (66.438, -82.3979)
  line L259 (66.438, -82.3979) -> (66.438, -83.5176)
  line L260 (66.438, -83.5176) -> (65.6767, -83.5176)
  line L261 (65.6767, -83.5176) -> (65.6767, -80.4676)
  line L262 (65.6767, -80.4676) -> (66.9027, -80.4676)
  spline S133 degree 2 poles (66.9027, -80.4676) (67.1573, -80.4676) (67.5329, -80.5319) (67.6936, -80.6307) knots 0 0 0 1 2 2 2
  spline S134 degree 2 poles (67.6936, -80.6307) (67.8567, -80.7345) (68.0495, -81.0583) (68.0495, -81.3055) knots 0 0 0 1 2 2 2
  spline S135 degree 2 poles (68.0495, -81.3055) (68.0495, -81.654) (67.7331, -82.0915) (67.4687, -82.22) knots 0 0 0 1 2 2 2
  line L263 (67.4687, -82.22) -> (68.4944, -83.5176)
  spline S136 degree 2 poles (67.2635, -81.4019) (67.2635, -81.2857) (67.1746, -81.1201) (67.0732, -81.0756) knots 0 0 0 1 2 2 2
  spline S137 degree 2 poles (67.0732, -81.0756) (67.0015, -81.046) (66.8261, -81.0287) (66.6951, -81.0287) knots 0 0 0 1 2 2 2
  line L264 (66.6951, -81.0287) -> (66.438, -81.0287)
  line L265 (66.438, -81.0287) -> (66.438, -81.8492)
  line L266 (66.438, -81.8492) -> (66.658, -81.8492)
  spline S138 degree 2 poles (66.658, -81.8492) (66.8162, -81.8492) (67.0411, -81.8097) (67.1177, -81.7479) knots 0 0 0 1 2 2 2
  spline S139 degree 2 poles (67.1177, -81.7479) (67.1919, -81.6886) (67.2635, -81.5304) (67.2635, -81.4019) knots 0 0 0 1 2 2 2
  line L267 (70.2394, -83.5176) -> (68.5982, -83.5176)
  line L268 (68.5982, -83.5176) -> (68.5982, -82.9862)
  line L269 (68.5982, -82.9862) -> (69.0357, -82.9862)
  line L270 (69.0357, -82.9862) -> (69.0357, -80.999)
  line L271 (69.0357, -80.999) -> (68.5982, -80.999)
  line L272 (68.5982, -80.999) -> (68.5982, -80.4676)
  line L273 (68.5982, -80.4676) -> (70.2394, -80.4676)
  line L274 (70.2394, -80.4676) -> (70.2394, -80.999)
  line L275 (70.2394, -80.999) -> (69.8019, -80.999)
  line L276 (69.8019, -80.999) -> (69.8019, -82.9862)
  line L277 (69.8019, -82.9862) -> (70.2394, -82.9862)
  line L278 (70.2394, -82.9862) -> (70.2394, -83.5176)
  line L279 (72.7901, -81.0484) -> (71.5098, -81.0484)
  line L280 (71.5098, -81.0484) -> (71.5098, -81.6243)
  line L281 (71.5098, -81.6243) -> (72.6888, -81.6243)
  line L282 (72.6888, -81.6243) -> (72.6888, -82.2052)
  line L283 (72.6888, -82.2052) -> (71.5098, -82.2052)
  line L284 (71.5098, -82.2052) -> (71.5098, -83.5176)
  line L285 (71.5098, -83.5176) -> (70.7485, -83.5176)
  line L286 (70.7485, -83.5176) -> (70.7485, -80.4676)
  line L287 (70.7485, -80.4676) -> (72.7901, -80.4676)
  line L288 (72.7901, -80.4676) -> (72.7901, -81.0484)
  line L289 (73.7714, -83.5176) -> (73.7714, -81.0484)
  line L290 (73.7714, -81.0484) -> (72.8692, -81.0484)
  line L291 (72.8692, -81.0484) -> (72.8692, -80.4676)
  line L292 (72.8692, -80.4676) -> (75.4397, -80.4676)
  line L293 (75.4397, -80.4676) -> (75.4397, -81.0484)
  line L294 (75.4397, -81.0484) -> (74.5376, -81.0484)
  line L295 (74.5376, -81.0484) -> (74.5376, -83.5176)
  line L296 (74.5376, -83.5176) -> (73.7714, -83.5176)
  spline S140 degree 2 poles (78.2969, -83.5769) (77.6098, -83.5769) (76.8041, -82.7465) (76.8041, -81.9951) knots 0 0 0 1 2 2 2
  spline S141 degree 2 poles (76.8041, -81.9951) (76.8041, -81.2709) (77.6123, -80.4083) (78.2994, -80.4083) knots 0 0 0 1 2 2 2
  spline S142 degree 2 poles (78.2994, -80.4083) (78.4798, -80.4083) (78.7715, -80.4503) (78.9049, -80.4849) knots 0 0 0 1 2 2 2
  spline S143 degree 2 poles (78.9049, -80.4849) (79.0088, -80.517) (79.2534, -80.6233) (79.3301, -80.6629) knots 0 0 0 1 2 2 2
  line L297 (79.3301, -80.6629) -> (79.3301, -81.3895)
  line L298 (79.3301, -81.3895) -> (79.2534, -81.3895)
  spline S144 degree 2 poles (79.2534, -81.3895) (79.1966, -81.3401) (79.0285, -81.2017) (78.9222, -81.1374) knots 0 0 0 1 2 2 2
  spline S145 degree 2 poles (78.9222, -81.1374) (78.816, -81.0707) (78.5614, -80.9792) (78.4205, -80.9792) knots 0 0 0 1 2 2 2
  spline S146 degree 2 poles (78.4205, -80.9792) (78.2549, -80.9792) (77.9806, -81.083) (77.8545, -81.214) knots 0 0 0 1 2 2 2